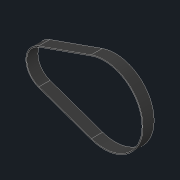
# Autodesk Inventor part: belt5
Saved by Autodesk Inventor 2022 (Build 260153000, 153)
## iProperties
Created: 2021-08-06
Part Number: belt5
Material: ゴム
Document SubType Name: Modeling
Designer: yuta0
Density: 0.93 g/cm^3
Appearance: ゴム - 黒
購入先: ミスミ
在庫数: 0.0
Author: yuta0
Autodesk Inventor part; units mm, degrees
ref_plane "YZ Plane" through (0, 0, 0) normal (1, 0, 0) x (0, 1, 0)
ref_plane "XZ Plane" through (0, 0, 0) normal (0, 1, 0) x (-1, 0, 0)
ref_plane "XY Plane" through (0, 0, 0) normal (0, 0, 1) x (1, 0, 0)
sketch "スケッチ1" plane through (0, 0, 0) normal (0, 0, 1) x (1, 0, 0)
  arc A0 (-5.5703, 15.7556) -> (-5.5703, -15.7556) centre (0, 0) ccw
  arc A1 (41.5411, -32.4115) -> (41.5411, 32.4115) centre (53, 0) ccw
  line L0 (-5.5703, 15.7556) -> (41.5411, 32.4115)
  line L1 (-5.5703, -15.7556) -> (41.5411, -32.4115)
  line L2 (41.4015, 32.8065) -> (-5.7099, 16.1506)
  arc A2 (-5.7099, 16.1506) -> (-5.7099, -16.1506) centre (0, 0) ccw
  line L3 (-5.7099, -16.1506) -> (41.4015, -32.8065)
  arc A3 (41.4015, -32.8065) -> (41.4015, 32.8065) centre (53, 0) ccw
  line L4 (41.6681, 32.0523) -> (-5.4433, 15.3964)
  arc A4 (-5.4433, 15.3964) -> (-5.4433, -15.3964) centre (0, 0) ccw
  line L5 (-5.4433, -15.3964) -> (41.6681, -32.0523)
  arc A5 (41.6681, -32.0523) -> (41.6681, 32.0523) centre (53, 0) ccw
  dimension "d6" = 33.4225
  dimension "d7" = 68.7549
  dimension "d8" = 53
  dimension "d11" = 0.419
  dimension "d12" = 0.8
  constraints: 12 end point, 12 point on circle, 6 centre point, 4 tangent, 1 coincident, 1 horizontal alignment, 6 other
  measures "d6" diameter of A0
  measures "d7" diameter of A1
  measures "d8" distance of A1.centre A0.centre
  measures "d11" distance between parallel lines of L0 L2
  measures "d12" distance between parallel lines of L2 L4
extrude "押し出し1" add sketch "スケッチ1" along normal mid plane 10 contours L0 A1 L1 A0 | A3 L3 A2 L2
